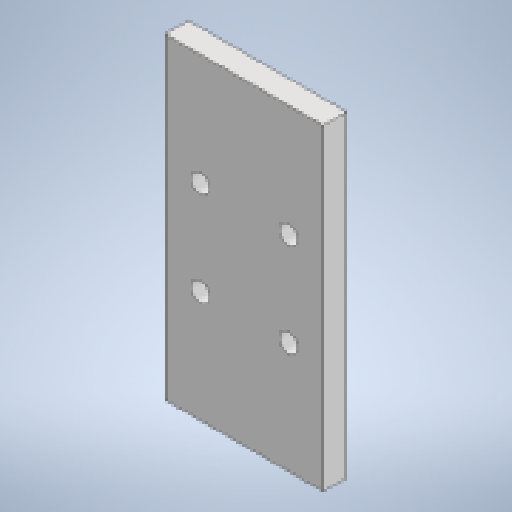
# Autodesk Inventor part: фанера_каретка
Saved by Autodesk Inventor 2023.1 (Build 271208000, 208)
## iProperties
Created: 2026-01-04
Part Number: фанера_каретка
Material: Типовые
Document SubType Name: Modeling
Designer: DELL
Density: 1 g/cm^3
Appearance: По умолчанию
Author: DELL
Autodesk Inventor part; units mm, degrees
ref_plane "YZ Plane" through (0, 0, 0) normal (1, 0, 0) x (0, 1, 0)
ref_plane "XZ Plane" through (0, 0, 0) normal (0, 1, 0) x (-1, 0, 0)
ref_plane "XY Plane" through (0, 0, 0) normal (0, 0, 1) x (1, 0, 0)
sketch "Эскиз1" plane through (0, 0, 0) normal (0, 0, 1) x (1, 0, 0)
  circle A0 centre (-7.5, -6.95) radius 1.5 construction
  circle A1 centre (7.5, -6.95) radius 1.5 construction
  circle A2 centre (7.5, -22.95) radius 1.5 construction
  circle A3 centre (-7.5, -22.95) radius 1.5 construction
  circle A4 centre (-7.5, -6.95) radius 1.6
  circle A5 centre (7.5, -6.95) radius 1.6
  circle A6 centre (7.5, -22.95) radius 1.6
  circle A7 centre (-7.5, -22.95) radius 1.6
  line L0 (9, 4.1) -> (-9, 4.1) construction
  line L1 (9, -34) -> (-9, -34) construction
  line L2 (-13.5, 12.05) -> (13.5, 12.05)
  line L3 (13.5, 12.05) -> (13.5, -41.95)
  line L4 (13.5, -41.95) -> (-13.5, -41.95)
  line L5 (-13.5, -41.95) -> (-13.5, 12.05)
  line L6 (-7.5, -6.95) -> (-7.5, 12.05) construction
  line L7 (-7.5, -22.95) -> (-7.5, -41.95) construction
  point P0 (0, 0)
  dimension "d0" = 3.2
  dimension "d1" = 3.2
  dimension "d2" = 3.2
  dimension "d3" = 3.2
  dimension "d4" = 6
  dimension "d5" = 6
  dimension "d8" = 54
  constraints: 12 end point, 4 centre point, 4 coincident, 3 point on line, 2 parallel, 2 perpendicular, 1 collinear, 1 horizontal
  measures "d0" diameter of A4
  measures "d1" diameter of A5
  measures "d2" diameter of A6
  measures "d3" diameter of A7
  measures "d4" distance from line of L3 A5.centre
  measures "d5" distance from line of L5 A0.centre
  measures "d8" distance between parallel lines of L4 L2
extrude "Выдавливание1" add sketch "Эскиз1" along normal blind 4
